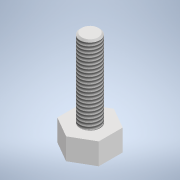
# Autodesk Inventor part: Pieza2
Saved by Autodesk Inventor 2020.3 (Build 243373010, 373A)
## iProperties
Created: 2020-11-12
Part Number: Pieza2
Material: Acero inoxidable, pulido
Document SubType Name: Modeling
Designer: codig
Density: 8 g/cm^3
Appearance: Inoxidable - Pulido
Author: codig
Autodesk Inventor part; units mm, degrees
ref_plane "YZ Plane" through (0, 0, 0) normal (1, 0, 0) x (0, 1, 0)
ref_plane "XZ Plane" through (0, 0, 0) normal (0, 1, 0) x (-1, 0, 0)
ref_plane "XY Plane" through (0, 0, 0) normal (0, 0, 1) x (1, 0, 0)
sketch "Boceto1" plane through (0, 0, 0) normal (0, 1, 0) x (-1, 0, 0)
  line L0 (106.25, -96.3916) -> (100, -92.7831)
  line L1 (100, -92.7831) -> (93.75, -96.3916)
  line L2 (93.75, -96.3916) -> (93.75, -103.6084)
  line L3 (93.75, -103.6084) -> (100, -107.2169)
  line L4 (100, -107.2169) -> (106.25, -103.6084)
  line L5 (106.25, -103.6084) -> (106.25, -96.3916)
  point P0 (0, 0)
  constraints: 12 end point, 3 parallel, 1 vertical
extrude "Extrusión1" add sketch "Boceto1" along normal blind 6.5
sketch "Boceto3" plane through (0, 6.5, 0) normal (0, 1, 0) x (1, 0, 0)
  circle A0 centre (-100, 100) radius 3
  point P0 (0, 0)
  constraints: 1 centre point
extrude "Extrusión2" add sketch "Boceto3" along normal blind 23.5
chamfer "Chaflán1" distance 0.5 angle 45 1 edges at (-103, 30, -100)
thread "Rosca1" size "M6x1" class "6g" standard "ISO Metric profile" full length
